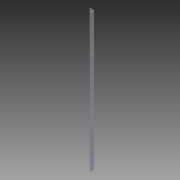
# Autodesk Inventor part: L-Frame
Saved by Autodesk Inventor 2015 (Build 190159000, 159)
## iProperties
Created: 2015-01-10
Part Number: L-Frame
Material: Aluminum 6061
Document SubType Name: Modeling
Designer: Chandler Willoughby
Density: 2.7 g/cm^3
Appearance: Aluminum - Flat
Author: Chandler Willoughby
Autodesk Inventor part; units mm, degrees
ref_plane "YZ Plane" through (0, 0, 0) normal (1, 0, 0) x (0, 1, 0)
ref_plane "XZ Plane" through (0, 0, 0) normal (0, 1, 0) x (-1, 0, 0)
ref_plane "XY Plane" through (0, 0, 0) normal (0, 0, 1) x (1, 0, 0)
sketch "Sketch1" plane through (0, 0, 0) normal (0, 1, 0) x (-1, 0, 0)
  line L0 (0, 0) -> (3.175, 0)
  line L1 (3.175, 0) -> (3.175, -47.625)
  line L2 (3.175, -47.625) -> (50.8, -47.625)
  line L3 (50.8, -47.625) -> (50.8, -50.8)
  line L4 (50.8, -50.8) -> (0, -50.8)
  line L5 (0, -50.8) -> (0, 0)
  dimension "d0" = 3.175
  dimension "d1" = 47.625
  dimension "d2" = 47.625
  dimension "d3" = 3.175
  dimension "d4" = 50.8
  dimension "d5" = 50.8
  constraints: 12 end point, 4 perpendicular, 1 horizontal
  measures "d0" distance of L0.start L0.end
  measures "d1" distance of L0.end L1.end
  measures "d2" distance of L1.end L2.end
  measures "d3" distance of L2.end L3.end
  measures "d4" distance of L3.end L4.end
  measures "d5" distance of L4.end L0.start
extrude "Extrusion1" add sketch "Sketch1" along normal blind 1828.8
body "Solid1"
